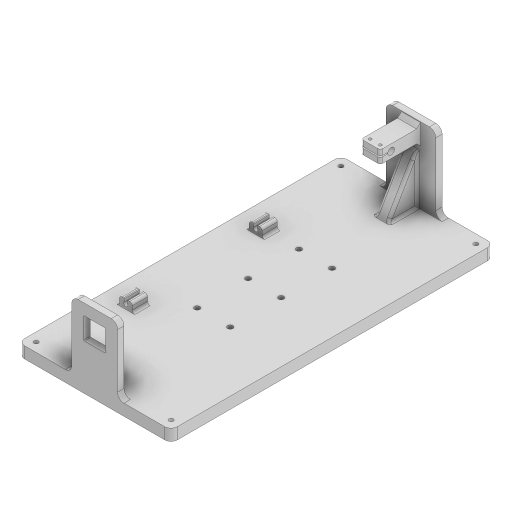
# Autodesk Inventor part: Enclosure base
Saved by Autodesk Inventor 2023 (Build 270158000, 158)
## iProperties
Created: 2026-05-19
Part Number: Enclosure base
Material: Generic
Document SubType Name: Modeling
Designer: ferrerx
Density: 1 g/cm^3
Appearance: Default
Author: ferrerx
Autodesk Inventor part; units mm, degrees
ref_plane "YZ Plane" through (0, 0, 0) normal (1, 0, 0) x (0, 1, 0)
ref_plane "XZ Plane" through (0, 0, 0) normal (0, 1, 0) x (-1, 0, 0)
ref_plane "XY Plane" through (0, 0, 0) normal (0, 0, 1) x (1, 0, 0)
sketch "Sketch1" plane through (0, 0, 0) normal (0, 1, 0) x (-1, 0, 0)
  line L0 (-60, 126.75) -> (60, 126.75)
  line L1 (60, 126.75) -> (60, -126.75)
  line L2 (60, -126.75) -> (-60, -126.75)
  line L3 (-60, -126.75) -> (-60, 126.75)
  line L4 (-60, 126.75) -> (60, -126.75) construction
  line L5 (60, 126.75) -> (-60, -126.75) construction
  line L6 (-13, 33.25) -> (13, 33.25) construction
  line L7 (13, 33.25) -> (13, -46.75) construction
  line L8 (13, -46.75) -> (-13, -46.75) construction
  line L9 (-13, -46.75) -> (-13, 33.25) construction
  line L10 (-13, 33.25) -> (13, -46.75) construction
  line L11 (13, 33.25) -> (-13, -46.75) construction
  circle A0 centre (13, 33.25) radius 2.05
  circle A1 centre (-13, 33.25) radius 2.05
  circle A2 centre (-13, -46.75) radius 2.05
  circle A3 centre (13, -46.75) radius 2.05
  circle A4 centre (-13, -6.75) radius 2.05
  circle A5 centre (13, -6.75) radius 2.05
  point P0 (0, 0)
  point P1 (0, -6.75)
  dimension "d0" = 26
  dimension "d1" = 80
  dimension "d3" = 4.1
  dimension "d4" = 4.1
  dimension "d5" = 4.1
  dimension "d6" = 4.1
  dimension "d7" = 4.1
  dimension "d8" = 4.1
  dimension "d15" = 120
  dimension "d16" = 80
  dimension "d17" = 93.5
  constraints: 24 end point, 6 centre point, 6 midpoint, 4 coincident, 4 parallel, 2 horizontal, 2 perpendicular
  measures "d0" distance of L7.end L8.end
  measures "d1" distance of L8.end L6.start
  measures "d3" diameter of A3
  measures "d4" diameter of A2
  measures "d5" diameter of A1
  measures "d6" diameter of A0
  measures "d7" diameter of A4
  measures "d8" diameter of A5
  measures "d15" distance of L1.end L2.end
  measures "d16" distance between parallel lines of L2 L8
  measures "d17" distance between parallel lines of L6 L0
extrude "Extrusion1" add sketch "Sketch1" along normal blind 7
sketch "Sketch2" plane through (0, 0, 0) normal (0, -1, 0) x (1, 0, 0)
  line L0 (60, -126.75) -> (-60, -126.75) projected
  line L1 (-60, 126.75) -> (60, 126.75)
  line L2 (60, 126.75) -> (60, -126.75)
  line L3 (60, -126.75) -> (-60, -126.75)
  line L4 (-60, -126.75) -> (-60, 126.75)
  line L5 (-60, 126.75) -> (60, -126.75) construction
  line L6 (60, 126.75) -> (-60, -126.75) construction
  point P0 (0, 0)
  constraints: 12 end point, 2 midpoint, 2 parallel, 1 horizontal, 1 perpendicular
extrude "Extrusion2" add sketch "Sketch2" along normal blind 2
sketch "Sketch3" plane through (0, 7, 0) normal (0, 1, 0) x (1, 0, 0)
  line L0 (-7.5, 50) -> (7.5, 50)
  line L1 (7.5, 50) -> (7.5, 65)
  line L2 (7.5, 65) -> (-7.5, 65)
  line L3 (-7.5, 65) -> (-7.5, 50)
  line L4 (-7.5, 50) -> (7.5, 65) construction
  line L5 (7.5, 50) -> (-7.5, 65) construction
  line L6 (0, 0) -> (0, 57.5) construction
  line L7 (-60, 126.75) -> (-60, -126.75) projected
  dimension "d18" = 15
  dimension "d19" = 15
  dimension "d22" = 50
  constraints: 14 end point, 3 parallel, 2 midpoint, 1 horizontal, 1 perpendicular
  measures "d18" distance between parallel lines of L2 L0
  measures "d19" distance of L0.start L0.end
  measures "d22" distance from line of L6.start L0
extrude "Extrusion3" [suppressed]
sketch "Sketch4" plane through (-10, 7, -65) normal (-1, 0, 0) x (0, 0, 1)
  line L0 (15, 60) -> (0, 60) projected
  line L1 (15, 60) -> (40, 60)
  line L2 (40, 60) -> (40, 50)
  line L3 (40, 50) -> (15, 50)
  line L4 (15, 50) -> (15, 60)
  point P0 (65, -7)
  dimension "d23" = 25
  dimension "d24" = 10
  constraints: 8 end point, 2 parallel, 1 horizontal, 1 perpendicular
  measures "d23" distance of L2.end L3.end
  measures "d24" distance between parallel lines of L3 L1
extrude "Extrusion4" [suppressed]
sketch "Sketch5" plane through (0, 7, 0) normal (0, 1, 0) x (1, 0, 0)
  line L0 (18.25, -126.75) -> (-18.25, -126.75) construction
  line L1 (-18.25, -126.75) -> (-18.25, -68.604) construction
  line L2 (-18.25, -68.604) -> (18.25, -68.604) construction
  line L3 (18.25, -68.604) -> (18.25, -126.75) construction
  line L4 (0, 0) -> (0, -126.75) construction
  line L5 (18.25, -126.75) -> (60, -126.75)
  line L6 (60, 126.75) -> (60, -126.75) projected
  line L7 (60, -126.75) -> (60, 126.75)
  line L8 (60, 126.75) -> (-60, 126.75)
  line L9 (-60, 126.75) -> (-60, -126.75) projected
  line L10 (18.25, -126.75) -> (18.25, -121.75)
  line L11 (18.25, -121.75) -> (55, -121.75)
  line L12 (55, -121.75) -> (55, 121.75)
  line L13 (55, 121.75) -> (-5, 121.75)
  line L14 (60, 126.75) -> (-60, 126.75) projected
  line L15 (0, 126.75) -> (60, 126.75)
  line L16 (-18.25, -68.604) -> (-18.25, -126.75) construction
  line L17 (-18.25, -126.75) -> (-60, -126.75)
  line L18 (-60, 126.75) -> (-60, -126.75)
  line L19 (-60, -126.75) -> (-60, 126.75)
  line L20 (-18.25, -126.75) -> (-18.25, -121.75)
  line L21 (-18.25, -121.75) -> (-55, -121.75)
  line L22 (-55, -121.75) -> (-55, 121.75)
  line L23 (-55, 121.75) -> (-5, 121.75)
  line L24 (0, 126.75) -> (-60, 126.75)
  dimension "d27" = 36.5
  dimension "d28" = 5
  dimension "d29" = 5
  dimension "d30" = 5
  constraints: 44 end point, 3 equal length, 3 horizontal, 3 perpendicular, 3 symmetric about line, 2 midpoint, 2 point on line, 1 vertical
  measures "d27" distance between parallel lines of L1 L3
  measures "d28" distance between parallel lines of L8 L13
  measures "d29" distance between parallel lines of L6 L12
  measures "d30" distance between parallel lines of L5 L11
extrude "Extrusion5" add sketch "Sketch5" along normal blind 70
sketch "Sketch7" plane through (-55, 7, -121.75) normal (0, 0, 1) x (1, 0, 0)
  line L0 (36.75, 0) -> (73.25, 0) projected
  line L1 (55, 0) -> (55, 51) construction
  line L2 (47.5, 56) -> (62.5, 56)
  line L3 (62.5, 56) -> (62.5, 46)
  line L4 (62.5, 46) -> (47.5, 46)
  line L5 (47.5, 46) -> (47.5, 56)
  line L6 (47.5, 56) -> (62.5, 46) construction
  line L7 (62.5, 56) -> (47.5, 46) construction
  point P0 (55, -7)
  dimension "d39" = 15
  dimension "d40" = 51
  dimension "d41" = 10
  constraints: 14 end point, 4 midpoint, 2 parallel, 1 horizontal, 1 perpendicular, 1 vertical
  measures "d39" distance of L2.start L2.end
  measures "d40" distance of point (55, 0) L1.end
  measures "d41" distance of L2.end L3.end
extrude "Extrusion6" add sketch "Sketch7" along normal blind 31.546
sketch "Sketch8" plane through (7.5, 53, -121.75) normal (1, 0, 0) x (0, 0, -1)
  line L0 (-31.546, 0) -> (-31.546, 10) projected
  line L1 (-31.546, 5) -> (-23.046, 5) construction
  circle A0 centre (-23.046, 5) radius 2.55
  line L2 (-32.3937, 5.5) -> (-24.877, 5.5)
  line L3 (-24.877, 5.5) -> (-24.877, 4.5)
  line L4 (-24.877, 4.5) -> (-32.3937, 4.5)
  line L5 (-32.3937, 4.5) -> (-32.3937, 5.5)
  line L6 (-32.3937, 5.5) -> (-24.877, 4.5) construction
  line L7 (-24.877, 5.5) -> (-32.3937, 4.5) construction
  point P0 (-121.75, -53)
  point P1 (-28.6353, 5)
  point P2 (-25.5465, 4.5)
  point P3 (-25.5465, 5.5)
  dimension "d44" = 5.1
  dimension "d45" = 8.5
  dimension "d46" = 1
  constraints: 14 end point, 3 midpoint, 2 horizontal, 2 parallel, 1 centre point, 1 coincident, 1 perpendicular, 1 point on line
  measures "d44" diameter of A0
  measures "d45" distance of L1.start L1.end
  measures "d46" distance between parallel lines of L2 L4
extrude "Extrusion7" cut sketch "Sketch8" against normal blind 20
sketch "Sketch9" plane through (-7.5, 63, -121.75) normal (0, 1, 0) x (1, 0, 0)
  circle A0 centre (11.5, -28.046) radius 1.1
  line L0 (15, -31.546) -> (0, -31.546) projected
  line L1 (7.5, -31.546) -> (7.5, 0) construction
  line L2 (-47.5, 0) -> (62.5, 0) projected
  line L3 (15, 0) -> (15, -31.546) projected
  circle A1 centre (3.5, -28.046) radius 1.1
  point P0 (7.5, -121.75)
  dimension "d49" = 2.2
  dimension "d50" = 3.5
  dimension "d51" = 3.5
  constraints: 2 centre point, 2 end point, 2 midpoint, 1 symmetric about line, 1 other
  measures "d49" diameter of A0
  measures "d50" distance from line of L3 A0.centre
  measures "d51" distance from line of L0 A0.centre
extrude "Extrusion8" cut sketch "Sketch9" against normal blind 20
sketch "Sketch10" plane through (-7.5, 53, -121.75) normal (0, -1, 0) x (1, 0, 0)
  circle A0 centre (3.5, 28.046) radius 1.1 projected
  circle A1 centre (3.5, 28.046) radius 1.6
  circle A2 centre (11.5, 28.046) radius 1.1 projected
  circle A3 centre (11.5, 28.046) radius 1.6
  point P0 (7.5, 121.75)
  dimension "d54" = 3.2
  dimension "d55" = 3.2
  constraints: 2 centre point, 2 coincident
  measures "d54" diameter of A1
  measures "d55" diameter of A3
extrude "Extrusion9" cut sketch "Sketch10" against normal blind 4
sketch "Sketch11" plane through (0, 77, 0) normal (0, 1, 0) x (1, 0, 0)
  line L0 (-60, 126.75) -> (60, 126.75) projected
  line L1 (-19.5, 126.75) -> (-19.5, 121.75)
  line L2 (-55, 121.75) -> (55, 121.75) projected
  line L3 (-19.5, 126.75) -> (-60, 126.75)
  line L4 (-60, -126.75) -> (-60, 126.75) projected
  line L5 (-60, 126.75) -> (-60, -126.75)
  line L6 (-60, -126.75) -> (-18.25, -126.75)
  line L7 (60, -126.75) -> (-60, -126.75) projected
  line L8 (-18.25, -121.75) -> (-55, -121.75)
  line L9 (-55, -121.75) -> (-55, 121.75)
  line L10 (-55, 121.75) -> (-19.5, 121.75)
  line L11 (-18.25, -121.75) -> (-18.25, -126.75)
  line L12 (-18.25, -126.75) -> (-18.25, -121.75) projected
  line L13 (0, 126.75) -> (0, -126.75) construction
  line L14 (19.5, 126.75) -> (19.5, 121.75)
  line L15 (19.5, 126.75) -> (60, 126.75)
  line L16 (60, -126.75) -> (60, 126.75)
  line L17 (60, 126.75) -> (60, -126.75)
  line L18 (60, -126.75) -> (18.25, -126.75)
  line L19 (18.25, -121.75) -> (55, -121.75)
  line L20 (55, -121.75) -> (55, 121.75)
  line L21 (55, 121.75) -> (19.5, 121.75)
  line L22 (18.25, -121.75) -> (18.25, -126.75)
  line L23 (18.25, -126.75) -> (18.25, -121.75)
  point P0 (0, 0)
  point P1 (55, 121.75)
  point P2 (18.25, -126.75)
  point P3 (19.5, 121.75)
  point P4 (-55, 121.75)
  dimension "d58" = 40.5
  constraints: 38 end point, 9 symmetric about line, 3 collinear, 3 point on line, 2 midpoint, 2 perpendicular, 1 horizontal, 1 vertical
  measures "d58" distance between parallel lines of L4 L1
extrude "Extrusion10" cut sketch "Sketch11" against normal up to surface (70 mm away) contours L0 L1 L2 L9 L8 L11 L6 L4 | L0 L16 L7 L22 L19 L20 L2 L14
fillet "Fillet1" radius 5 4 edges at (-60, 2.5, -126.75) (-60, 2.5, 126.75) (60, 2.5, 126.75) (60, 2.5, -126.75)
thicken "Thicken1" operation cut thickness 10.5 both sides no extend neighbours no toward (0, -1, 0) faces at (6.5, 77, -123.4167)
sketch "Sketch12" plane through (0, 0, 0) normal (1, 0, 0) x (0, 1, 0)
  line L0 (7, -121.75) -> (66.5, -121.75) projected
  line L1 (47, -121.75) -> (7, -98.656)
  line L2 (7, -121.75) -> (7, 121.75) projected
  line L3 (7, -121.75) -> (47, -121.75)
  point P0 (0, 0)
  dimension "d66" = 30
  dimension "d67" = 40
  constraints: 4 end point, 2 point on line, 1 horizontal
  measures "d66" angle of L0 L1
  measures "d67" distance of L0.start L1.start
extrude "Extrusion11" add sketch "Sketch12" along normal mid plane 10
chamfer "Chamfer1" distance 3 angle 45 2 edges at (0, 53, -121.75) (0, 63, -121.75)
fillet "Fillet2" radius 2 6 edges at (-5, 7, -110.203) (-5, 27, -121.75) (-5, 27, -110.203) (5, 27, -110.203) (5, 7, -110.203) (5, 27, -121.75)
sketch "Sketch13" plane through (0, 7, 0) normal (0, 1, 0) x (1, 0, 0)
  line L0 (55, -126.75) -> (-55, -126.75) projected
  line L1 (18, -126.75) -> (-18, -126.75)
  line L2 (-18, -126.75) -> (-18, -121.75)
  line L3 (-18, -121.75) -> (18, -121.75)
  line L4 (18, -121.75) -> (18, -126.75)
  point P0 (0, 0)
  dimension "d74" = 5
  dimension "d75" = 18
  dimension "d76" = 18
  constraints: 8 end point, 2 parallel, 1 horizontal, 1 perpendicular, 1 point on line
  measures "d74" distance of L3.end L1.start
  measures "d75" distance from line of point (0, 0) L2
  measures "d76" distance from line of point (0, 0) L4
extrude "Extrusion12" add sketch "Sketch13" along normal blind 52.5
sketch "Sketch14" plane through (-55, -2, 126.75) normal (0, 0, 1) x (1, 0, 0)
  line L0 (46.5, 52.8) -> (63.5, 52.8)
  line L1 (63.5, 52.8) -> (63.5, 35.8)
  line L2 (63.5, 35.8) -> (46.5, 35.8)
  line L3 (46.5, 35.8) -> (46.5, 52.8)
  line L4 (46.5, 52.8) -> (63.5, 35.8) construction
  line L5 (63.5, 52.8) -> (46.5, 35.8) construction
  line L6 (55, 44.3) -> (55, 0) construction
  line L7 (0, 0) -> (110, 0) projected
  line L8 (0, 9) -> (37, 9) projected
  point P0 (55, 2)
  dimension "d79" = 17
  dimension "d80" = 17
  dimension "d81" = 26.8
  constraints: 14 end point, 3 midpoint, 2 parallel, 1 horizontal, 1 perpendicular, 1 vertical
  measures "d79" distance of L0.end L1.end
  measures "d80" distance of L1.end L2.end
  measures "d81" distance between parallel lines of L8 L2
extrude "Extrusion13" cut sketch "Sketch14" against normal blind 59.5
fillet "Fillet3" radius 0.5 4 edges at (8.5, 50.8, 124.25) (8.5, 33.8, 124.25) (-8.5, 33.8, 124.25) (-8.5, 50.8, 124.25)
sketch "Sketch15" plane through (0, 7, 0) normal (0, 1, 0) x (1, 0, 0)
  line L0 (53, -119.75) -> (-53, -119.75) construction
  line L1 (-53, -119.75) -> (-53, 119.75) construction
  line L2 (-53, 119.75) -> (53, 119.75) construction
  line L3 (53, 119.75) -> (53, -119.75) construction
  line L4 (53, -119.75) -> (-53, 119.75) construction
  line L5 (-53, -119.75) -> (53, 119.75) construction
  line L6 (-60, -121.75) -> (-60, 121.75) projected
  line L7 (-55, -126.75) -> (-18, -126.75) projected
  circle A0 centre (-53, -119.75) radius 1.7
  circle A1 centre (-53, 119.75) radius 1.7
  circle A2 centre (53, 119.75) radius 1.7
  circle A3 centre (53, -119.75) radius 1.7
  point P0 (0, 0)
  dimension "d85" = 7
  dimension "d86" = 7
  dimension "d87" = 3.4
  dimension "d88" = 3.4
  dimension "d89" = 3.4
  dimension "d90" = 3.4
  constraints: 12 end point, 4 centre point, 4 coincident, 2 midpoint, 2 parallel, 1 horizontal, 1 perpendicular
  measures "d85" distance between parallel lines of L6 L1
  measures "d86" distance between parallel lines of L7 L0
  measures "d87" diameter of A0
  measures "d88" diameter of A1
  measures "d89" diameter of A2
  measures "d90" diameter of A3
extrude "Extrusion14" cut sketch "Sketch15" against normal blind 6
fillet "Fillet4" radius 5 8 edges at (-19.5, 66.5, -124.25) (19.5, 66.5, -124.25) (-18, 59.5, 124.25) (18, 59.5, 124.25) (-18, 7, 124.25) (18, 7, 124.25) (-19.5, 7, -124.25) (19.5, 7, -124.25)
fillet "Fillet5" radius 2 4 edges at (-7.5, 60.75, -90.204) (7.5, 60.75, -90.204) (-7.5, 55.25, -90.204) (7.5, 55.25, -90.204)
sketch "Sketch16" plane through (0, 7, 0) normal (0, 1, 0) x (1, 0, 0)
  line L0 (-35, 51.75) -> (-45, 51.75)
  line L1 (-45, 51.75) -> (-45, 39.75)
  line L2 (-45, 39.75) -> (-35, 39.75)
  line L3 (-35, 39.75) -> (-35, 51.75)
  line L4 (-35, 51.75) -> (-45, 39.75) construction
  line L5 (-45, 51.75) -> (-35, 39.75) construction
  line L6 (-35, -50.25) -> (-45, -50.25)
  line L7 (-45, -50.25) -> (-45, -62.25)
  line L8 (-45, -62.25) -> (-35, -62.25)
  line L9 (-35, -62.25) -> (-35, -50.25)
  line L10 (-35, -50.25) -> (-45, -62.25) construction
  line L11 (-45, -50.25) -> (-35, -62.25) construction
  line L12 (-60, -121.75) -> (-60, 121.75) projected
  line L13 (-55, 126.75) -> (-24.5, 126.75) projected
  point P0 (0, 0)
  point P1 (-40, 45.75)
  point P2 (-40, -56.25)
  dimension "d95" = 10
  dimension "d96" = 20
  dimension "d97" = 10
  dimension "d98" = 12
  dimension "d99" = 12
  dimension "d100" = 75
  dimension "d101" = 90
  constraints: 24 end point, 4 midpoint, 4 parallel, 2 horizontal, 2 perpendicular, 1 point on line
  measures "d95" distance of L1.end L2.end
  measures "d96" distance from line of L12 point (-40, 45.75)
  measures "d97" distance of L7.end L8.end
  measures "d98" distance of L6.end L7.end
  measures "d99" distance of L0.end L1.end
  measures "d100" distance between parallel lines of L13 L0
  measures "d101" distance between parallel lines of L6 L2
extrude "Extrusion15" add sketch "Sketch16" along normal blind 7
sketch "Sketch17" plane through (-45, 7, 62.25) normal (0, 0, 1) x (1, 0, 0)
  line L0 (0, 7) -> (10, 7) projected
  line L1 (5, 7) -> (5, 3.5) construction
  circle A0 centre (5, 3.5) radius 1.6
  line L2 (3.65, 2.8476) -> (6.35, 2.8476)
  line L3 (6.35, 2.8476) -> (6.35, 7.3524)
  line L4 (6.35, 7.3524) -> (3.65, 7.3524)
  line L5 (3.65, 7.3524) -> (3.65, 2.8476)
  line L6 (3.65, 2.8476) -> (6.35, 7.3524) construction
  line L7 (6.35, 2.8476) -> (3.65, 7.3524) construction
  point P0 (45, -7)
  point P1 (5, 5.1)
  point P2 (3.65, 4.3588)
  point P3 (6.35, 4.3588)
  dimension "d104" = 3.2
  dimension "d105" = 3.5
  dimension "d106" = 2.7
  constraints: 14 end point, 3 midpoint, 2 parallel, 1 coincident, 1 horizontal, 1 perpendicular, 1 point on line, 1 vertical, 3 other
  measures "d105" distance from line of L0 point (5, 3.5)
  measures "d106" distance of L3.end L4.end
extrude "Extrusion16" cut sketch "Sketch17" against normal blind 119
fillet "Fillet6" radius 2 8 edges at (-45, 7, -45.75) (-45, 7, 56.25) (-45, 14, -45.75) (-35, 14, -45.75) (-45, 14, 56.25) (-35, 14, 56.25) (-35, 7, 56.25) (-35, 7, -45.75)
fillet "Fillet7" radius 0.5 4 edges at (-38.65, 14, 56.25) (-41.35, 14, 56.25) (-38.65, 14, -45.75) (-41.35, 14, -45.75)
equation "\"d4\" = d3"
equation "\"d5\" = d4"
equation "\"d6\" = d3"
equation "\"d7\" = d3"
equation "\"d8\" = d3"
equation "\"d75\" = d76"
equation "\"d97\" = d95"
body "Solid1"
